Autodesk Fusion 360 part; units mm, degrees
(part 3 of 4)
  point P31 (-40.625, 1.496)
  point P32 (-27.125, 9.2902)
  point P33 (-18.125, 9.2902)
  point P34 (-13.625, 1.496)
  point P35 (-22.625, 1.496)
  point P36 (-9.125, 9.2902)
  point P37 (-0.125, 9.2902)
  point P38 (4.375, 1.496)
  point P39 (-4.625, 1.496)
  point P40 (8.875, 9.2902)
  point P41 (17.875, 9.2902)
  point P42 (22.375, 1.496)
  point P43 (13.375, 1.496)
  point P44 (-153.125, 25.1672)
  point P45 (-144.125, 25.1672)
  point P46 (-139.625, 17.373)
  point P47 (-148.625, 17.373)
  point P48 (-135.125, 25.1672)
  point P49 (-126.125, 25.1672)
  point P50 (-121.625, 17.373)
  point P51 (-130.625, 17.373)
  point P52 (-117.125, 25.1672)
  point P53 (-108.125, 25.1672)
  point P54 (-103.625, 17.373)
  point P55 (-112.625, 17.373)
  point P56 (-99.125, 25.1672)
  point P57 (-90.125, 25.1672)
  point P58 (-85.625, 17.373)
  point P59 (-94.625, 17.373)
  point P60 (-81.125, 25.1672)
  point P61 (-72.125, 25.1672)
  point P62 (-67.625, 17.373)
  point P63 (-76.625, 17.373)
  point P64 (-63.125, 25.1672)
  point P65 (-54.125, 25.1672)
  point P66 (-49.625, 17.373)
  point P67 (-58.625, 17.373)
  point P68 (-45.125, 25.1672)
  point P69 (-36.125, 25.1672)
  point P70 (-31.625, 17.373)
  point P71 (-40.625, 17.373)
  point P72 (-27.125, 25.1672)
  point P73 (-18.125, 25.1672)
  point P74 (-13.625, 17.373)
  point P75 (-22.625, 17.373)
  point P76 (-9.125, 25.1672)
  point P77 (-0.125, 25.1672)
  point P78 (4.375, 17.373)
  point P79 (-4.625, 17.373)
  point P80 (8.875, 25.1672)
  point P81 (17.875, 25.1672)
  point P82 (22.375, 17.373)
  point P83 (13.375, 17.373)
  point P84 (-153.125, 41.0442)
  point P85 (-144.125, 41.0442)
  point P86 (-139.625, 33.25)
  point P87 (-148.625, 33.25)
  point P88 (-135.125, 41.0442)
  point P89 (-126.125, 41.0442)
  point P90 (-121.625, 33.25)
  point P91 (-130.625, 33.25)
  point P92 (-117.125, 41.0442)
  point P93 (-108.125, 41.0442)
  point P94 (-103.625, 33.25)
  point P95 (-112.625, 33.25)
  point P96 (-99.125, 41.0442)
  point P97 (-90.125, 41.0442)
  point P98 (-85.625, 33.25)
  point P99 (-94.625, 33.25)
  point P100 (-63.125, 41.0442)
  point P101 (-54.125, 41.0442)
  point P102 (-49.625, 33.25)
  point P103 (-58.625, 33.25)
  point P104 (-45.125, 41.0442)
  point P105 (-36.125, 41.0442)
  point P106 (-31.625, 33.25)
  point P107 (-40.625, 33.25)
  point P108 (-27.125, 41.0442)
  point P109 (-18.125, 41.0442)
  point P110 (-13.625, 33.25)
  point P111 (-22.625, 33.25)
  point P112 (-9.125, 41.0442)
  point P113 (-0.125, 41.0442)
  point P114 (4.375, 33.25)
  point P115 (-4.625, 33.25)
  point P116 (8.875, 41.0442)
  point P117 (17.875, 41.0442)
  point P118 (22.375, 33.25)
  point P119 (13.375, 33.25)
  point P120 (-153.125, 56.9212)
  point P121 (-144.125, 56.9212)
  point P122 (-139.625, 49.127)
  point P123 (-148.625, 49.127)
  point P124 (-135.125, 56.9212)
  point P125 (-126.125, 56.9212)
  point P126 (-121.625, 49.127)
  point P127 (-130.625, 49.127)
  point P128 (-117.125, 56.9212)
  point P129 (-108.125, 56.9212)
  point P130 (-103.625, 49.127)
  point P131 (-112.625, 49.127)
  point P132 (-99.125, 56.9212)
  point P133 (-90.125, 56.9212)
  point P134 (-85.625, 49.127)
  point P135 (-94.625, 49.127)
  point P136 (-81.125, 56.9212)
  point P137 (-72.125, 56.9212)
  point P138 (-67.625, 49.127)
  point P139 (-76.625, 49.127)
  point P140 (-63.125, 56.9212)
  point P141 (-54.125, 56.9212)
  point P142 (-49.625, 49.127)
  point P143 (-58.625, 49.127)
  point P144 (-45.125, 56.9212)
  point P145 (-36.125, 56.9212)
  point P146 (-31.625, 49.127)
  point P147 (-40.625, 49.127)
  point P148 (-27.125, 56.9212)
  point P149 (-18.125, 56.9212)
  point P150 (-13.625, 49.127)
  point P151 (-22.625, 49.127)
  point P152 (-9.125, 56.9212)
  point P153 (-0.125, 56.9212)
  point P154 (4.375, 49.127)
  point P155 (-4.625, 49.127)
  point P156 (8.875, 56.9212)
  point P157 (17.875, 56.9212)
  point P158 (22.375, 49.127)
  point P159 (13.375, 49.127)
  point P160 (-153.125, 72.7982)
  point P161 (-144.125, 72.7982)
  point P162 (-139.625, 65.004)
  point P163 (-148.625, 65.004)
  point P164 (-135.125, 72.7982)
  point P165 (-126.125, 72.7982)
  point P166 (-121.625, 65.004)
  point P167 (-130.625, 65.004)
  point P168 (-117.125, 72.7982)
  point P169 (-108.125, 72.7982)
  point P170 (-103.625, 65.004)
  point P171 (-112.625, 65.004)
  point P172 (-99.125, 72.7982)
  point P173 (-90.125, 72.7982)
  point P174 (-85.625, 65.004)
  point P175 (-94.625, 65.004)
  point P176 (-81.125, 72.7982)
  point P177 (-72.125, 72.7982)
  point P178 (-67.625, 65.004)
  point P179 (-76.625, 65.004)
  point P180 (-63.125, 72.7982)
  point P181 (-54.125, 72.7982)
  point P182 (-49.625, 65.004)
  point P183 (-58.625, 65.004)
  point P184 (-45.125, 72.7982)
  point P185 (-36.125, 72.7982)
  point P186 (-31.625, 65.004)
  point P187 (-40.625, 65.004)
  point P188 (-27.125, 72.7982)
  point P189 (-18.125, 72.7982)
  point P190 (-13.625, 65.004)
  point P191 (-22.625, 65.004)
  point P192 (-9.125, 72.7982)
  point P193 (-0.125, 72.7982)
  point P194 (4.375, 65.004)
  point P195 (-4.625, 65.004)
  point P196 (8.875, 72.7982)
  point P197 (17.875, 72.7982)
  point P198 (22.375, 65.004)
  point P199 (13.375, 65.004)
  point P200 (-153.125, 88.6752)
  point P201 (-144.125, 88.6752)
  point P202 (-139.625, 80.881)
  point P203 (-148.625, 80.881)
  point P204 (-135.125, 88.6752)
  point P205 (-126.125, 88.6752)
  point P206 (-121.625, 80.881)
  point P207 (-130.625, 80.881)
  point P208 (-117.125, 88.6752)
  point P209 (-108.125, 88.6752)
  point P210 (-103.625, 80.881)
  point P211 (-112.625, 80.881)
  point P212 (-99.125, 88.6752)
  point P213 (-90.125, 88.6752)
  point P214 (-85.625, 80.881)
  point P215 (-94.625, 80.881)
  point P216 (-81.125, 88.6752)
  point P217 (-72.125, 88.6752)
  point P218 (-67.625, 80.881)
  point P219 (-76.625, 80.881)
  point P220 (-63.125, 88.6752)
  point P221 (-54.125, 88.6752)
  point P222 (-49.625, 80.881)
  point P223 (-58.625, 80.881)
  point P224 (-45.125, 88.6752)
  point P225 (-36.125, 88.6752)
  point P226 (-31.625, 80.881)
  point P227 (-40.625, 80.881)
  point P228 (-27.125, 88.6752)
  point P229 (-18.125, 88.6752)
  point P230 (-13.625, 80.881)
  point P231 (-22.625, 80.881)
  point P232 (-9.125, 88.6752)
  point P233 (-0.125, 88.6752)
  point P234 (4.375, 80.881)
  point P235 (-4.625, 80.881)
  point P236 (8.875, 88.6752)
  point P237 (17.875, 88.6752)
  point P238 (22.375, 80.881)
  point P239 (13.375, 80.881)
  dimension "d110" = 2
  dimension "d111" = 150.75
  dimension "d112" = 2
  dimension "d113" = 2
  dimension "d115" = 150.75
  dimension "d116" = 6
  dimension "d118" = 3.5
  dimension "d119" = 3.5
  dimension "d120" = 3.5
  dimension "d121" = 3.5
  dimension "d122" = 2
  dimension "d123" = 2
  dimension "d124" = 2
  dimension "d125" = 2
  dimension "d126" = 2
  dimension "d129" = 18
  dimension "d130" = 15.877
  dimension "d131" = 2
  constraint horizontal L16
  constraint vertical L17
  constraint coincident L11.end L12.start
  constraint horizontal L18
  constraint vertical L19
  constraint horizontal L20
  constraint vertical L21
  constraint horizontal L22
  constraint vertical L23
  constraint horizontal L24
  constraint vertical L25
  constraint horizontal L26
  constraint vertical L27
  constraint vertical L28
  constraint vertical L29
  constraint horizontal L30
  constraint vertical L31
  constraint coincident L19 L29.end
  constraint coincident L14 L29.end
  constraint horizontal L32
  constraint vertical L33
  constraint vertical L34
  constraint horizontal L35
  constraint coincident L12.end L13.start
  constraint horizontal L36
  constraint vertical L37
  constraint horizontal L38
  constraint vertical L39
  constraint coincident L38 L40.end
  constraint perpendicular L38 L40
  constraint horizontal L1481
  constraint vertical L1482
  constraint horizontal L1483
  constraint vertical L1484
  constraint perpendicular L18 L1485
  measures "d110" distance of L17.end L18.end
  measures "d111" distance of L19.end L10.end
  measures "d112" distance of L19.end L24.end
  measures "d113" distance of L23.end L26.end
  measures "d115" distance of L11.end L36.end
  measures "d116" distance of L11.end L38.end
  measures "d118" distance of P0 L46
  measures "d119" distance of P1 L52
  measures "d120" distance of P2 L58
  measures "d121" distance of P3 L64
  measures "d122" distance of L42 L63
  measures "d123" distance of L55 L64
  measures "d124" distance of L41 L56
  measures "d125" distance of L46 L49
  measures "d126" distance of L48 L57
  measures "d131" distance of L29.end L1483.end
extrude "Extrude18" cut sketch "Sketch14" against normal blind 2 contours L38 L263 L264 L267 L268 L269 L272 | L19 L29 L258 L262 L271 L1485 | L38 L233 L234 L235 L238 L247 L249 | L19 L29 L500 L505 L506 L510 L520 | L38 L239 L240 L243 L244 L245 L248 | L19 L29 L498 L502 L511 | L38 L209 L210 L211 L214 L223 L225 | L19 L29 L714 L718 L727 | L19 L29 L716 L721 L722 L726 L736 | L38 L215 L216 L219 L220 L221 L224 | L19 L29 L958 L967 L1483 | L19 L29 L956 L961 L962 L966 L976 | L38 L185 L186 L187 L190 L199 L201 | L960 L964 L965 L968 L1483 | L38 L191 L192 L195 L196 L197 L200 | L931 L934 L943 L945 L1483 | L38 L161 L162 L163 L166 L175 L177 | L936 L940 L941 L944 L1483 | L38 L167 L168 L171 L172 L173 L176 | L907 L910 L919 L921 L1483 | L38 L137 L138 L139 L142 L151 L153 | L912 L916 L917 L920 L1483 | L38 L143 L144 L147 L148 L149 L152 | L883 L886 L895 L897 L1483 | L38 L113 L114 L115 L118 L127 L129 | L27 L31 L40 L72 L75 L77 | L38 L65 L66 L67 L70 L79 L81 | L888 L892 L893 L896 L1483 | L38 L119 L120 L123 L124 L125 L128 | L27 L31 L312 L315 L317 | L27 L31 L309 L313 L314 L318 L328 | L38 L95 L96 L99 L100 L101 L104 | L859 L862 L871 L873 L1483 | L38 L89 L90 L91 L94 L103 L105 | L27 L31 L552 L555 L557 | L27 L31 L549 L553 L554 L558 L568 | L864 L868 L869 L872 L1483 | L27 L31 L768 L773 L1483 | L27 L31 L765 L769 L770 L774 L784 | L835 L838 L847 L849 L1483 | L840 L844 L845 L848 L1483 | L763 L766 L775 L777 L1483 | L811 L814 L823 L825 L1483 | L792 L796 L797 L800 L1483 | L816 L820 L821 L824 L1483 | L787 L790 L799 L801 L1483 | L41 L42 L43 L44 L45 L46 | L47 L48 L49 L50 L51 L52 | L53 L54 L55 L56 L57 L58 | L59 L60 L61 L62 L63 L64 | L305 L306 L307 L310 L319 L321 | L322 L323 L324 L325 L326 L327 | L329 L330 L331 L334 L343 L345 | L332 L333 L337 L338 L342 L352 | L335 L336 L339 L340 L341 L344 | L346 L347 L348 L349 L350 L351 | L353 L354 L355 L358 L367 L369 | L356 L357 L361 L362 L366 L376 | L359 L360 L363 L364 L365 L368 | L370 L371 L372 L373 L374 L375 | L377 L378 L379 L382 L391 L393 | L380 L381 L385 L386 L390 L400 | L383 L384 L387 L388 L389 L392 | L394 L395 L396 L397 L398 L399 | L401 L402 L403 L406 L415 L417 | L404 L405 L409 L410 L414 L424 | L407 L408 L411 L412 L413 L416 | L418 L419 L420 L421 L422 L423 | L425 L426 L427 L430 L439 L441 | L428 L429 L433 L434 L438 L448 | L431 L432 L435 L436 L437 L440 | L442 L443 L444 L445 L446 L447 | L449 L450 L451 L454 L463 L465 | L452 L453 L457 L458 L462 L472 | L455 L456 L459 L460 L461 L464 | L466 L467 L468 L469 L470 L471 | L473 L474 L475 L478 L487 L489 | L476 L477 L481 L482 L486 L496 | L479 L480 L483 L484 L485 L488 | L490 L491 L492 L493 L494 L495 | L503 L504 L507 L508 L509 L512 | L545 L546 L547 L550 L559 L561 | L562 L563 L564 L565 L566 L567 | L569 L570 L571 L574 L583 L585 | L572 L573 L577 L578 L582 L592 | L575 L576 L579 L580 L581 L584 | L586 L587 L588 L589 L590 L591 | L593 L594 L595 L598 L607 L609 | L596 L597 L601 L602 L606 L616 | L599 L600 L603 L604 L605 L608 | L610 L611 L612 L613 L614 L615 | L617 L618 L619 L622 L631 L633 | L620 L621 L625 L626 L630 L640 | L623 L624 L627 L628 L629 L632 | L634 L635 L636 L637 L638 L639 | L641 L642 L643 L646 L655 L657 | L644 L645 L649 L650 L654 L664 | L647 L648 L651 L652 L653 L656 | L658 L659 L660 L661 L662 L663 | L665 L666 L667 L670 L679 L681 | L668 L669 L673 L674 L678 L688 | L671 L672 L675 L676 L677 L680 | L682 L683 L684 L685 L686 L687 | L689 L690 L691 L694 L703 L705 | L692 L693 L697 L698 L702 L712 | L695 L696 L699 L700 L701 L704 | L706 L707 L708 L709 L710 L711 | L719 L720 L723 L724 L725 L728 | L778 L779 L780 L781 L782 L783 | L788 L789 L793 L794 L798 L808 | L802 L803 L804 L805 L806 L807 | L812 L813 L817 L818 L822 L832 | L826 L827 L828 L829 L830 L831 | L836 L837 L841 L842 L846 L856 | L850 L851 L852 L853 L854 L855 | L860 L861 L865 L866 L870 L880 | L874 L875 L876 L877 L878 L879 | L884 L885 L889 L890 L894 L904 | L898 L899 L900 L901 L902 L903 | L908 L909 L913 L914 L918 L928 | L922 L923 L924 L925 L926 L927 | L932 L933 L937 L938 L942 L952 | L946 L947 L948 L949 L950 L951 bodies 2
sketch "Sketch15" plane through (0, 0, 0) normal (1, 0, 0) x (0, 0, -1)
  line L0 (85, 3) -> (85, 3.5)
  arc A0 (86, 4.5) -> (85, 3.5) centre (86, 3.5) ccw
  line L1 (86, 4.5) -> (104, 4.5)
  arc A1 (105, 3.5) -> (104, 4.5) centre (104, 3.5) ccw
  line L2 (105, 3.5) -> (105, 3)
  arc A2 (104, 2) -> (105, 3) centre (104, 3) ccw
  line L3 (104, 2) -> (86, 2)
  arc A3 (85, 3) -> (86, 2) centre (86, 3) ccw
  line L4 (29, 2) -> (11, 2)
  arc A4 (10, 3) -> (11, 2) centre (11, 3) ccw
  line L5 (10, 3) -> (10, 3.5)
  arc A5 (11, 4.5) -> (10, 3.5) centre (11, 3.5) ccw
  line L6 (11, 4.5) -> (29, 4.5)
  arc A6 (30, 3.5) -> (29, 4.5) centre (29, 3.5) ccw
  line L7 (30, 3.5) -> (30, 3)
  arc A7 (29, 2) -> (30, 3) centre (29, 3) ccw
  line L8 (10.25, 71) -> (114.75, 71)
  line L9 (114.75, 71) -> (114.75, 85)
  line L10 (114.75, 85) -> (-2, 85)
  line L11 (-2, 85) -> (-2, 0)
  line L12 (-2, 0) -> (114.75, 0)
  line L13 (114.75, 0) -> (114.75, 60)
  line L14 (114.75, 60) -> (10.25, 60)
  line L15 (10.25, 60) -> (10.25, 71)
  line L16 (114.75, 0) -> (-2, 0)
  line L17 (-2, 0) -> (-2, 6)
  line L18 (-2, 6) -> (114.75, 6)
  line L19 (114.75, 6) -> (114.75, 0)
  line L20 (-2, 6) -> (0, 6)
  line L21 (0, 6) -> (0, 60)
  line L22 (0, 60) -> (-2, 60)
  line L23 (-2, 60) -> (-2, 6)
  line L24 (-2, 60) -> (114.75, 60)
  line L25 (114.75, 60) -> (114.75, 58)
  line L26 (114.75, 58) -> (-2, 58)
  line L27 (-2, 58) -> (-2, 60)
  line L28 (114.75, 58) -> (112.75, 58)
  line L29 (112.75, 58) -> (112.75, 6)
  line L30 (112.75, 6) -> (114.75, 6)
  line L31 (114.75, 6) -> (114.75, 58)
  line L32 (112.75, 32) -> (112.75, 6)
  line L33 (112.75, 6) -> (56.375, 6)
  line L34 (59.875, 34.0207) -> (56.375, 36.0415)
  line L35 (56.375, 36.0415) -> (52.875, 34.0207)
  line L36 (52.875, 34.0207) -> (52.875, 29.9793)
  line L37 (52.875, 29.9793) -> (56.375, 27.9585)
  line L38 (56.375, 27.9585) -> (59.875, 29.9793)
  line L39 (59.875, 29.9793) -> (59.875, 34.0207)
  line L40 (68.875, 34.0207) -> (65.375, 36.0415)
  line L41 (65.375, 36.0415) -> (61.875, 34.0207)
  line L42 (61.875, 34.0207) -> (61.875, 29.9793)
  line L43 (61.875, 29.9793) -> (65.375, 27.9585)
  line L44 (65.375, 27.9585) -> (68.875, 29.9793)
  line L45 (68.875, 29.9793) -> (68.875, 34.0207)
  line L46 (64.375, 41.815) -> (60.875, 43.8357)
  line L47 (60.875, 43.8357) -> (57.375, 41.815)
  line L48 (57.375, 41.815) -> (57.375, 37.7735)
  line L49 (57.375, 37.7735) -> (60.875, 35.7528)
  line L50 (60.875, 35.7528) -> (64.375, 37.7735)
  line L51 (64.375, 37.7735) -> (64.375, 41.815)
  line L52 (55.375, 41.815) -> (51.875, 43.8357)
  line L53 (51.875, 43.8357) -> (48.375, 41.815)
  line L54 (48.375, 41.815) -> (48.375, 37.7735)
  line L55 (48.375, 37.7735) -> (51.875, 35.7528)
  line L56 (51.875, 35.7528) -> (55.375, 37.7735)
  line L57 (55.375, 37.7735) -> (55.375, 41.815)
  line L58 (1.375, 10.061) -> (-2.125, 12.0817)
  line L59 (10.375, 6.0195) -> (10.375, 10.061)
  line L60 (6.875, 12.0817) -> (3.375, 10.061)
  line L61 (3.375, 6.0195) -> (6.875, 3.9988)
  line L62 (5.875, 2.2667) -> (2.375, 4.2875)
  line L63 (1.375, 6.0195) -> (1.375, 10.061)
  line L64 (11.375, -3.7955) -> (14.875, -1.7747)
  line L65 (-5.625, 10.061) -> (-5.625, 6.0195)
  line L66 (6.875, 3.9988) -> (10.375, 6.0195)
  line L67 (2.375, 4.2875) -> (-1.125, 2.2667)
  line L68 (-2.125, 3.9988) -> (1.375, 6.0195)
  line L69 (10.375, 10.061) -> (6.875, 12.0817)
  line L70 (-5.625, 6.0195) -> (-2.125, 3.9988)
  line L71 (2.375, -3.7955) -> (5.875, -1.7747)
  line L72 (11.375, 4.2875) -> (7.875, 2.2667)
  line L73 (3.375, 10.061) -> (3.375, 6.0195)
  line L74 (-1.125, -1.7747) -> (2.375, -3.7955)
  line L75 (7.875, -1.7747) -> (11.375, -3.7955)
  line L76 (7.875, 2.2667) -> (7.875, -1.7747)
  line L77 (5.875, -1.7747) -> (5.875, 2.2667)
  line L78 (-1.125, 2.2667) -> (-1.125, -1.7747)
  line L79 (14.875, -1.7747) -> (14.875, 2.2667)
  line L80 (-2.125, 12.0817) -> (-5.625, 10.061)
  line L81 (14.875, 2.2667) -> (11.375, 4.2875)
  line L82 (19.375, 10.061) -> (15.875, 12.0817)
  line L83 (28.375, 6.0195) -> (28.375, 10.061)
  line L84 (24.875, 12.0817) -> (21.375, 10.061)
  line L85 (21.375, 6.0195) -> (24.875, 3.9988)
  line L86 (23.875, 2.2667) -> (20.375, 4.2875)
  line L87 (19.375, 6.0195) -> (19.375, 10.061)
  line L88 (29.375, -3.7955) -> (32.875, -1.7747)
  line L89 (12.375, 10.061) -> (12.375, 6.0195)
  line L90 (24.875, 3.9988) -> (28.375, 6.0195)
  line L91 (20.375, 4.2875) -> (16.875, 2.2667)
  line L92 (15.875, 3.9988) -> (19.375, 6.0195)
  line L93 (28.375, 10.061) -> (24.875, 12.0817)
  line L94 (12.375, 6.0195) -> (15.875, 3.9988)
  line L95 (20.375, -3.7955) -> (23.875, -1.7747)
  line L96 (29.375, 4.2875) -> (25.875, 2.2667)
  line L97 (21.375, 10.061) -> (21.375, 6.0195)
  line L98 (16.875, -1.7747) -> (20.375, -3.7955)
  line L99 (25.875, -1.7747) -> (29.375, -3.7955)
  line L100 (25.875, 2.2667) -> (25.875, -1.7747)
  line L101 (23.875, -1.7747) -> (23.875, 2.2667)
  line L102 (16.875, 2.2667) -> (16.875, -1.7747)
  line L103 (32.875, -1.7747) -> (32.875, 2.2667)
  line L104 (15.875, 12.0817) -> (12.375, 10.061)
  line L105 (32.875, 2.2667) -> (29.375, 4.2875)
  line L106 (37.375, 10.061) -> (33.875, 12.0817)
  line L107 (46.375, 6.0195) -> (46.375, 10.061)
  line L108 (42.875, 12.0817) -> (39.375, 10.061)
  line L109 (39.375, 6.0195) -> (42.875, 3.9988)
  line L110 (41.875, 2.2667) -> (38.375, 4.2875)
  line L111 (37.375, 6.0195) -> (37.375, 10.061)
  line L112 (47.375, -3.7955) -> (50.875, -1.7747)
  line L113 (30.375, 10.061) -> (30.375, 6.0195)
  line L114 (42.875, 3.9988) -> (46.375, 6.0195)
  line L115 (38.375, 4.2875) -> (34.875, 2.2667)
  line L116 (33.875, 3.9988) -> (37.375, 6.0195)
  line L117 (46.375, 10.061) -> (42.875, 12.0817)
  line L118 (30.375, 6.0195) -> (33.875, 3.9988)
  line L119 (38.375, -3.7955) -> (41.875, -1.7747)
  line L120 (47.375, 4.2875) -> (43.875, 2.2667)
  line L121 (39.375, 10.061) -> (39.375, 6.0195)
  line L122 (34.875, -1.7747) -> (38.375, -3.7955)
  line L123 (43.875, -1.7747) -> (47.375, -3.7955)
  line L124 (43.875, 2.2667) -> (43.875, -1.7747)
  line L125 (41.875, -1.7747) -> (41.875, 2.2667)
  line L126 (34.875, 2.2667) -> (34.875, -1.7747)
  line L127 (50.875, -1.7747) -> (50.875, 2.2667)
  line L128 (33.875, 12.0817) -> (30.375, 10.061)
  line L129 (50.875, 2.2667) -> (47.375, 4.2875)
  line L130 (55.375, 10.061) -> (51.875, 12.0817)
  line L131 (64.375, 6.0195) -> (64.375, 10.061)
  line L132 (60.875, 12.0817) -> (57.375, 10.061)
  line L133 (57.375, 6.0195) -> (60.875, 3.9988)
  line L134 (59.875, 2.2667) -> (56.375, 4.2875)
  line L135 (55.375, 6.0195) -> (55.375, 10.061)
  line L136 (65.375, -3.7955) -> (68.875, -1.7747)
  line L137 (48.375, 10.061) -> (48.375, 6.0195)
  line L138 (60.875, 3.9988) -> (64.375, 6.0195)
  line L139 (56.375, 4.2875) -> (52.875, 2.2667)
  line L140 (51.875, 3.9988) -> (55.375, 6.0195)
  line L141 (64.375, 10.061) -> (60.875, 12.0817)
  line L142 (48.375, 6.0195) -> (51.875, 3.9988)
  line L143 (56.375, -3.7955) -> (59.875, -1.7747)
  line L144 (65.375, 4.2875) -> (61.875, 2.2667)
  line L145 (57.375, 10.061) -> (57.375, 6.0195)
  line L146 (52.875, -1.7747) -> (56.375, -3.7955)
  line L147 (61.875, -1.7747) -> (65.375, -3.7955)
  line L148 (61.875, 2.2667) -> (61.875, -1.7747)
  line L149 (59.875, -1.7747) -> (59.875, 2.2667)
  line L150 (52.875, 2.2667) -> (52.875, -1.7747)
  line L151 (68.875, -1.7747) -> (68.875, 2.2667)
  line L152 (51.875, 12.0817) -> (48.375, 10.061)
  line L153 (68.875, 2.2667) -> (65.375, 4.2875)
  line L154 (73.375, 10.061) -> (69.875, 12.0817)
  line L155 (82.375, 6.0195) -> (82.375, 10.061)
  line L156 (78.875, 12.0817) -> (75.375, 10.061)
  line L157 (75.375, 6.0195) -> (78.875, 3.9988)
  line L158 (77.875, 2.2667) -> (74.375, 4.2875)
  line L159 (73.375, 6.0195) -> (73.375, 10.061)
  line L160 (83.375, -3.7955) -> (86.875, -1.7747)
  line L161 (66.375, 10.061) -> (66.375, 6.0195)
  line L162 (78.875, 3.9988) -> (82.375, 6.0195)
  line L163 (74.375, 4.2875) -> (70.875, 2.2667)
  line L164 (69.875, 3.9988) -> (73.375, 6.0195)
  line L165 (82.375, 10.061) -> (78.875, 12.0817)
  line L166 (66.375, 6.0195) -> (69.875, 3.9988)
  line L167 (74.375, -3.7955) -> (77.875, -1.7747)
  line L168 (83.375, 4.2875) -> (79.875, 2.2667)
  line L169 (75.375, 10.061) -> (75.375, 6.0195)
  line L170 (70.875, -1.7747) -> (74.375, -3.7955)
  line L171 (79.875, -1.7747) -> (83.375, -3.7955)
  line L172 (79.875, 2.2667) -> (79.875, -1.7747)
  line L173 (77.875, -1.7747) -> (77.875, 2.2667)
  line L174 (70.875, 2.2667) -> (70.875, -1.7747)
  line L175 (86.875, -1.7747) -> (86.875, 2.2667)
  line L176 (69.875, 12.0817) -> (66.375, 10.061)
  line L177 (86.875, 2.2667) -> (83.375, 4.2875)
  line L178 (91.375, 10.061) -> (87.875, 12.0817)
  line L179 (100.375, 6.0195) -> (100.375, 10.061)
  line L180 (96.875, 12.0817) -> (93.375, 10.061)
  line L181 (93.375, 6.0195) -> (96.875, 3.9988)
  line L182 (95.875, 2.2667) -> (92.375, 4.2875)
  line L183 (91.375, 6.0195) -> (91.375, 10.061)
  line L184 (101.375, -3.7955) -> (104.875, -1.7747)
  line L185 (84.375, 10.061) -> (84.375, 6.0195)
  line L186 (96.875, 3.9988) -> (100.375, 6.0195)
  line L187 (92.375, 4.2875) -> (88.875, 2.2667)
  line L188 (87.875, 3.9988) -> (91.375, 6.0195)
  line L189 (100.375, 10.061) -> (96.875, 12.0817)
  line L190 (84.375, 6.0195) -> (87.875, 3.9988)
  line L191 (92.375, -3.7955) -> (95.875, -1.7747)
  line L192 (101.375, 4.2875) -> (97.875, 2.2667)
  line L193 (93.375, 10.061) -> (93.375, 6.0195)
  line L194 (88.875, -1.7747) -> (92.375, -3.7955)
  line L195 (97.875, -1.7747) -> (101.375, -3.7955)
  line L196 (97.875, 2.2667) -> (97.875, -1.7747)
  line L197 (95.875, -1.7747) -> (95.875, 2.2667)
  line L198 (88.875, 2.2667) -> (88.875, -1.7747)
  line L199 (104.875, -1.7747) -> (104.875, 2.2667)
  line L200 (87.875, 12.0817) -> (84.375, 10.061)
  line L201 (104.875, 2.2667) -> (101.375, 4.2875)
  line L202 (109.375, 10.061) -> (105.875, 12.0817)
  line L203 (118.375, 6.0195) -> (118.375, 10.061)
  line L204 (114.875, 12.0817) -> (111.375, 10.061)
  line L205 (111.375, 6.0195) -> (114.875, 3.9988)
  line L206 (113.875, 2.2667) -> (110.375, 4.2875)
  line L207 (109.375, 6.0195) -> (109.375, 10.061)
  line L208 (119.375, -3.7955) -> (122.875, -1.7747)
  line L209 (102.375, 10.061) -> (102.375, 6.0195)
  line L210 (114.875, 3.9988) -> (118.375, 6.0195)
  line L211 (110.375, 4.2875) -> (106.875, 2.2667)
  line L212 (105.875, 3.9988) -> (109.375, 6.0195)
  line L213 (118.375, 10.061) -> (114.875, 12.0817)
  line L214 (102.375, 6.0195) -> (105.875, 3.9988)
  line L215 (110.375, -3.7955) -> (113.875, -1.7747)
  line L216 (119.375, 4.2875) -> (115.875, 2.2667)
  line L217 (111.375, 10.061) -> (111.375, 6.0195)
  line L218 (106.875, -1.7747) -> (110.375, -3.7955)
  line L219 (115.875, -1.7747) -> (119.375, -3.7955)
  line L220 (115.875, 2.2667) -> (115.875, -1.7747)
  line L221 (113.875, -1.7747) -> (113.875, 2.2667)
  line L222 (106.875, 2.2667) -> (106.875, -1.7747)
  line L223 (122.875, -1.7747) -> (122.875, 2.2667)
  line L224 (105.875, 12.0817) -> (102.375, 10.061)
  line L225 (122.875, 2.2667) -> (119.375, 4.2875)
  line L226 (1.375, 25.938) -> (-2.125, 27.9587)
  line L227 (10.375, 21.8965) -> (10.375, 25.938)
  line L228 (6.875, 27.9587) -> (3.375, 25.938)
  line L229 (3.375, 21.8965) -> (6.875, 19.8758)
  line L230 (5.875, 18.1437) -> (2.375, 20.1645)
  line L231 (1.375, 21.8965) -> (1.375, 25.938)
  line L232 (11.375, 12.0815) -> (14.875, 14.1023)
  line L233 (-5.625, 25.938) -> (-5.625, 21.8965)
  line L234 (6.875, 19.8758) -> (10.375, 21.8965)
  line L235 (2.375, 20.1645) -> (-1.125, 18.1437)
  line L236 (-2.125, 19.8758) -> (1.375, 21.8965)
  line L237 (10.375, 25.938) -> (6.875, 27.9587)
  line L238 (-5.625, 21.8965) -> (-2.125, 19.8758)
  line L239 (2.375, 12.0815) -> (5.875, 14.1023)
  line L240 (11.375, 20.1645) -> (7.875, 18.1437)
  line L241 (3.375, 25.938) -> (3.375, 21.8965)
  line L242 (-1.125, 14.1023) -> (2.375, 12.0815)
  line L243 (7.875, 14.1023) -> (11.375, 12.0815)
  line L244 (7.875, 18.1437) -> (7.875, 14.1023)
  line L245 (5.875, 14.1023) -> (5.875, 18.1437)
  line L246 (-1.125, 18.1437) -> (-1.125, 14.1023)
  line L247 (14.875, 14.1023) -> (14.875, 18.1437)
  line L248 (-2.125, 27.9587) -> (-5.625, 25.938)
  line L249 (14.875, 18.1437) -> (11.375, 20.1645)
  line L250 (19.375, 25.938) -> (15.875, 27.9587)
  line L251 (28.375, 21.8965) -> (28.375, 25.938)
  line L252 (24.875, 27.9587) -> (21.375, 25.938)
  line L253 (21.375, 21.8965) -> (24.875, 19.8758)
  line L254 (23.875, 18.1437) -> (20.375, 20.1645)
  line L255 (19.375, 21.8965) -> (19.375, 25.938)
  line L256 (29.375, 12.0815) -> (32.875, 14.1023)
  line L257 (12.375, 25.938) -> (12.375, 21.8965)
  line L258 (24.875, 19.8758) -> (28.375, 21.8965)
  line L259 (20.375, 20.1645) -> (16.875, 18.1437)
  line L260 (15.875, 19.8758) -> (19.375, 21.8965)
  line L261 (28.375, 25.938) -> (24.875, 27.9587)
  line L262 (12.375, 21.8965) -> (15.875, 19.8758)
  line L263 (20.375, 12.0815) -> (23.875, 14.1023)
  line L264 (29.375, 20.1645) -> (25.875, 18.1437)
  line L265 (21.375, 25.938) -> (21.375, 21.8965)
  line L266 (16.875, 14.1023) -> (20.375, 12.0815)
  line L267 (25.875, 14.1023) -> (29.375, 12.0815)
  line L268 (25.875, 18.1437) -> (25.875, 14.1023)
  line L269 (23.875, 14.1023) -> (23.875, 18.1437)
  line L270 (16.875, 18.1437) -> (16.875, 14.1023)
  line L271 (32.875, 14.1023) -> (32.875, 18.1437)
  line L272 (15.875, 27.9587) -> (12.375, 25.938)
  line L273 (32.875, 18.1437) -> (29.375, 20.1645)
  line L274 (37.375, 25.938) -> (33.875, 27.9587)
  line L275 (46.375, 21.8965) -> (46.375, 25.938)
  line L276 (42.875, 27.9587) -> (39.375, 25.938)
  line L277 (39.375, 21.8965) -> (42.875, 19.8758)
  line L278 (41.875, 18.1437) -> (38.375, 20.1645)
  line L279 (37.375, 21.8965) -> (37.375, 25.938)
  line L280 (47.375, 12.0815) -> (50.875, 14.1023)
  line L281 (30.375, 25.938) -> (30.375, 21.8965)
  line L282 (42.875, 19.8758) -> (46.375, 21.8965)
  line L283 (38.375, 20.1645) -> (34.875, 18.1437)
  line L284 (33.875, 19.8758) -> (37.375, 21.8965)
  line L285 (46.375, 25.938) -> (42.875, 27.9587)
  line L286 (30.375, 21.8965) -> (33.875, 19.8758)
  line L287 (38.375, 12.0815) -> (41.875, 14.1023)
  line L288 (47.375, 20.1645) -> (43.875, 18.1437)
  line L289 (39.375, 25.938) -> (39.375, 21.8965)
  line L290 (34.875, 14.1023) -> (38.375, 12.0815)
  line L291 (43.875, 14.1023) -> (47.375, 12.0815)
  line L292 (43.875, 18.1437) -> (43.875, 14.1023)
  line L293 (41.875, 14.1023) -> (41.875, 18.1437)
  line L294 (34.875, 18.1437) -> (34.875, 14.1023)
  line L295 (50.875, 14.1023) -> (50.875, 18.1437)
  line L296 (33.875, 27.9587) -> (30.375, 25.938)
  line L297 (50.875, 18.1437) -> (47.375, 20.1645)
  line L298 (55.375, 25.938) -> (51.875, 27.9587)
  line L299 (64.375, 21.8965) -> (64.375, 25.938)
  line L300 (60.875, 27.9587) -> (57.375, 25.938)
  line L301 (57.375, 21.8965) -> (60.875, 19.8758)
  line L302 (59.875, 18.1437) -> (56.375, 20.1645)
  line L303 (55.375, 21.8965) -> (55.375, 25.938)
  line L304 (65.375, 12.0815) -> (68.875, 14.1023)
  line L305 (48.375, 25.938) -> (48.375, 21.8965)
  line L306 (60.875, 19.8758) -> (64.375, 21.8965)
  line L307 (56.375, 20.1645) -> (52.875, 18.1437)
  line L308 (51.875, 19.8758) -> (55.375, 21.8965)
  line L309 (64.375, 25.938) -> (60.875, 27.9587)
  line L310 (48.375, 21.8965) -> (51.875, 19.8758)
  line L311 (56.375, 12.0815) -> (59.875, 14.1023)
  line L312 (65.375, 20.1645) -> (61.875, 18.1437)
  line L313 (57.375, 25.938) -> (57.375, 21.8965)
  line L314 (52.875, 14.1023) -> (56.375, 12.0815)
  line L315 (61.875, 14.1023) -> (65.375, 12.0815)
  line L316 (61.875, 18.1437) -> (61.875, 14.1023)
  line L317 (59.875, 14.1023) -> (59.875, 18.1437)
  line L318 (52.875, 18.1437) -> (52.875, 14.1023)
  line L319 (68.875, 14.1023) -> (68.875, 18.1437)
  line L320 (51.875, 27.9587) -> (48.375, 25.938)
  line L321 (68.875, 18.1437) -> (65.375, 20.1645)
  line L322 (73.375, 25.938) -> (69.875, 27.9587)
  line L323 (82.375, 21.8965) -> (82.375, 25.938)
  line L324 (78.875, 27.9587) -> (75.375, 25.938)
  line L325 (75.375, 21.8965) -> (78.875, 19.8758)
  line L326 (77.875, 18.1437) -> (74.375, 20.1645)
  line L327 (73.375, 21.8965) -> (73.375, 25.938)
  line L328 (83.375, 12.0815) -> (86.875, 14.1023)
  line L329 (66.375, 25.938) -> (66.375, 21.8965)
  line L330 (78.875, 19.8758) -> (82.375, 21.8965)
  line L331 (74.375, 20.1645) -> (70.875, 18.1437)
  line L332 (69.875, 19.8758) -> (73.375, 21.8965)
  line L333 (82.375, 25.938) -> (78.875, 27.9587)
  line L334 (66.375, 21.8965) -> (69.875, 19.8758)
  line L335 (74.375, 12.0815) -> (77.875, 14.1023)
  line L336 (83.375, 20.1645) -> (79.875, 18.1437)
  line L337 (75.375, 25.938) -> (75.375, 21.8965)
  line L338 (70.875, 14.1023) -> (74.375, 12.0815)
  line L339 (79.875, 14.1023) -> (83.375, 12.0815)
  line L340 (79.875, 18.1437) -> (79.875, 14.1023)
  line L341 (77.875, 14.1023) -> (77.875, 18.1437)
  line L342 (70.875, 18.1437) -> (70.875, 14.1023)
  line L343 (86.875, 14.1023) -> (86.875, 18.1437)
  line L344 (69.875, 27.9587) -> (66.375, 25.938)
  line L345 (86.875, 18.1437) -> (83.375, 20.1645)
  line L346 (91.375, 25.938) -> (87.875, 27.9587)
  line L347 (100.375, 21.8965) -> (100.375, 25.938)
  line L348 (96.875, 27.9587) -> (93.375, 25.938)
  line L349 (93.375, 21.8965) -> (96.875, 19.8758)
  line L350 (95.875, 18.1437) -> (92.375, 20.1645)
  line L351 (91.375, 21.8965) -> (91.375, 25.938)
  line L352 (101.375, 12.0815) -> (104.875, 14.1023)
  line L353 (84.375, 25.938) -> (84.375, 21.8965)
  line L354 (96.875, 19.8758) -> (100.375, 21.8965)
  line L355 (92.375, 20.1645) -> (88.875, 18.1437)
  line L356 (87.875, 19.8758) -> (91.375, 21.8965)
  line L357 (100.375, 25.938) -> (96.875, 27.9587)
  line L358 (84.375, 21.8965) -> (87.875, 19.8758)
  line L359 (92.375, 12.0815) -> (95.875, 14.1023)
  line L360 (101.375, 20.1645) -> (97.875, 18.1437)
  line L361 (93.375, 25.938) -> (93.375, 21.8965)
  line L362 (88.875, 14.1023) -> (92.375, 12.0815)
  line L363 (97.875, 14.1023) -> (101.375, 12.0815)
  line L364 (97.875, 18.1437) -> (97.875, 14.1023)
  line L365 (95.875, 14.1023) -> (95.875, 18.1437)
  line L366 (88.875, 18.1437) -> (88.875, 14.1023)
  line L367 (104.875, 14.1023) -> (104.875, 18.1437)
  line L368 (87.875, 27.9587) -> (84.375, 25.938)
  line L369 (104.875, 18.1437) -> (101.375, 20.1645)
  line L370 (109.375, 25.938) -> (105.875, 27.9587)
  line L371 (118.375, 21.8965) -> (118.375, 25.938)
  line L372 (114.875, 27.9587) -> (111.375, 25.938)
  line L373 (111.375, 21.8965) -> (114.875, 19.8758)
  line L374 (113.875, 18.1437) -> (110.375, 20.1645)
  line L375 (109.375, 21.8965) -> (109.375, 25.938)
  line L376 (119.375, 12.0815) -> (122.875, 14.1023)
  line L377 (102.375, 25.938) -> (102.375, 21.8965)
  line L378 (114.875, 19.8758) -> (118.375, 21.8965)
  line L379 (110.375, 20.1645) -> (106.875, 18.1437)
  line L380 (105.875, 19.8758) -> (109.375, 21.8965)
  line L381 (118.375, 25.938) -> (114.875, 27.9587)
  line L382 (102.375, 21.8965) -> (105.875, 19.8758)
  line L383 (110.375, 12.0815) -> (113.875, 14.1023)
  line L384 (119.375, 20.1645) -> (115.875, 18.1437)
  line L385 (111.375, 25.938) -> (111.375, 21.8965)
  line L386 (106.875, 14.1023) -> (110.375, 12.0815)
  line L387 (115.875, 14.1023) -> (119.375, 12.0815)
  line L388 (115.875, 18.1437) -> (115.875, 14.1023)
  line L389 (113.875, 14.1023) -> (113.875, 18.1437)
  line L390 (106.875, 18.1437) -> (106.875, 14.1023)
  line L391 (122.875, 14.1023) -> (122.875, 18.1437)
  line L392 (105.875, 27.9587) -> (102.375, 25.938)
  line L393 (122.875, 18.1437) -> (119.375, 20.1645)
  line L394 (1.375, 41.815) -> (-2.125, 43.8357)
  line L395 (10.375, 37.7735) -> (10.375, 41.815)
  line L396 (6.875, 43.8357) -> (3.375, 41.815)
  line L397 (3.375, 37.7735) -> (6.875, 35.7528)
  line L398 (5.875, 34.0207) -> (2.375, 36.0415)
  line L399 (1.375, 37.7735) -> (1.375, 41.815)
  line L400 (11.375, 27.9585) -> (14.875, 29.9793)
  line L401 (-5.625, 41.815) -> (-5.625, 37.7735)
  line L402 (6.875, 35.7528) -> (10.375, 37.7735)
  line L403 (2.375, 36.0415) -> (-1.125, 34.0207)
  line L404 (-2.125, 35.7528) -> (1.375, 37.7735)
  line L405 (10.375, 41.815) -> (6.875, 43.8357)
  line L406 (-5.625, 37.7735) -> (-2.125, 35.7528)
  line L407 (2.375, 27.9585) -> (5.875, 29.9793)
  line L408 (11.375, 36.0415) -> (7.875, 34.0207)
  line L409 (3.375, 41.815) -> (3.375, 37.7735)
  line L410 (-1.125, 29.9793) -> (2.375, 27.9585)
  line L411 (7.875, 29.9793) -> (11.375, 27.9585)
  line L412 (7.875, 34.0207) -> (7.875, 29.9793)
  line L413 (5.875, 29.9793) -> (5.875, 34.0207)
  line L414 (-1.125, 34.0207) -> (-1.125, 29.9793)
  line L415 (14.875, 29.9793) -> (14.875, 34.0207)
  line L416 (-2.125, 43.8357) -> (-5.625, 41.815)
  line L417 (14.875, 34.0207) -> (11.375, 36.0415)
  line L418 (19.375, 41.815) -> (15.875, 43.8357)
  line L419 (28.375, 37.7735) -> (28.375, 41.815)
  line L420 (24.875, 43.8357) -> (21.375, 41.815)
  line L421 (21.375, 37.7735) -> (24.875, 35.7528)
  line L422 (23.875, 34.0207) -> (20.375, 36.0415)
  line L423 (19.375, 37.7735) -> (19.375, 41.815)
  line L424 (29.375, 27.9585) -> (32.875, 29.9793)
  line L425 (12.375, 41.815) -> (12.375, 37.7735)
  line L426 (24.875, 35.7528) -> (28.375, 37.7735)
  line L427 (20.375, 36.0415) -> (16.875, 34.0207)
  line L428 (15.875, 35.7528) -> (19.375, 37.7735)
  line L429 (28.375, 41.815) -> (24.875, 43.8357)
  line L430 (12.375, 37.7735) -> (15.875, 35.7528)
  line L431 (20.375, 27.9585) -> (23.875, 29.9793)
  line L432 (29.375, 36.0415) -> (25.875, 34.0207)
  line L433 (21.375, 41.815) -> (21.375, 37.7735)
  line L434 (16.875, 29.9793) -> (20.375, 27.9585)
  line L435 (25.875, 29.9793) -> (29.375, 27.9585)
  line L436 (25.875, 34.0207) -> (25.875, 29.9793)
  line L437 (23.875, 29.9793) -> (23.875, 34.0207)
  line L438 (16.875, 34.0207) -> (16.875, 29.9793)
  line L439 (32.875, 29.9793) -> (32.875, 34.0207)
  line L440 (15.875, 43.8357) -> (12.375, 41.815)
  line L441 (32.875, 34.0207) -> (29.375, 36.0415)
  line L442 (37.375, 41.815) -> (33.875, 43.8357)
  line L443 (46.375, 37.7735) -> (46.375, 41.815)
  line L444 (42.875, 43.8357) -> (39.375, 41.815)
  line L445 (39.375, 37.7735) -> (42.875, 35.7528)
  line L446 (41.875, 34.0207) -> (38.375, 36.0415)
  line L447 (37.375, 37.7735) -> (37.375, 41.815)
  line L448 (47.375, 27.9585) -> (50.875, 29.9793)
  line L449 (30.375, 41.815) -> (30.375, 37.7735)
  line L450 (42.875, 35.7528) -> (46.375, 37.7735)
  line L451 (38.375, 36.0415) -> (34.875, 34.0207)
  line L452 (33.875, 35.7528) -> (37.375, 37.7735)
  line L453 (46.375, 41.815) -> (42.875, 43.8357)
  line L454 (30.375, 37.7735) -> (33.875, 35.7528)
  line L455 (38.375, 27.9585) -> (41.875, 29.9793)
  line L456 (47.375, 36.0415) -> (43.875, 34.0207)
  line L457 (39.375, 41.815) -> (39.375, 37.7735)
  line L458 (34.875, 29.9793) -> (38.375, 27.9585)
  line L459 (43.875, 29.9793) -> (47.375, 27.9585)
  line L460 (43.875, 34.0207) -> (43.875, 29.9793)
  line L461 (41.875, 29.9793) -> (41.875, 34.0207)
  line L462 (34.875, 34.0207) -> (34.875, 29.9793)
  line L463 (50.875, 29.9793) -> (50.875, 34.0207)
  line L464 (33.875, 43.8357) -> (30.375, 41.815)
  line L465 (50.875, 34.0207) -> (47.375, 36.0415)
  line L466 (73.375, 41.815) -> (69.875, 43.8357)
  line L467 (82.375, 37.7735) -> (82.375, 41.815)
  line L468 (78.875, 43.8357) -> (75.375, 41.815)
  line L469 (75.375, 37.7735) -> (78.875, 35.7528)
  line L470 (77.875, 34.0207) -> (74.375, 36.0415)
  line L471 (73.375, 37.7735) -> (73.375, 41.815)
  line L472 (83.375, 27.9585) -> (86.875, 29.9793)
  line L473 (66.375, 41.815) -> (66.375, 37.7735)
  line L474 (78.875, 35.7528) -> (82.375, 37.7735)
  line L475 (74.375, 36.0415) -> (70.875, 34.0207)
  line L476 (69.875, 35.7528) -> (73.375, 37.7735)
  line L477 (82.375, 41.815) -> (78.875, 43.8357)
  line L478 (66.375, 37.7735) -> (69.875, 35.7528)
  line L479 (74.375, 27.9585) -> (77.875, 29.9793)
  line L480 (83.375, 36.0415) -> (79.875, 34.0207)
  line L481 (75.375, 41.815) -> (75.375, 37.7735)
  line L482 (70.875, 29.9793) -> (74.375, 27.9585)
  line L483 (79.875, 29.9793) -> (83.375, 27.9585)
  line L484 (79.875, 34.0207) -> (79.875, 29.9793)
  line L485 (77.875, 29.9793) -> (77.875, 34.0207)
  line L486 (70.875, 34.0207) -> (70.875, 29.9793)
  line L487 (86.875, 29.9793) -> (86.875, 34.0207)
  line L488 (69.875, 43.8357) -> (66.375, 41.815)
  line L489 (86.875, 34.0207) -> (83.375, 36.0415)
  line L490 (91.375, 41.815) -> (87.875, 43.8357)
  line L491 (100.375, 37.7735) -> (100.375, 41.815)
  line L492 (96.875, 43.8357) -> (93.375, 41.815)
  line L493 (93.375, 37.7735) -> (96.875, 35.7528)
  line L494 (95.875, 34.0207) -> (92.375, 36.0415)
  line L495 (91.375, 37.7735) -> (91.375, 41.815)
  line L496 (101.375, 27.9585) -> (104.875, 29.9793)
  line L497 (84.375, 41.815) -> (84.375, 37.7735)
  line L498 (96.875, 35.7528) -> (100.375, 37.7735)
  line L499 (92.375, 36.0415) -> (88.875, 34.0207)
  line L500 (87.875, 35.7528) -> (91.375, 37.7735)
  line L501 (100.375, 41.815) -> (96.875, 43.8357)
  line L502 (84.375, 37.7735) -> (87.875, 35.7528)
  line L503 (92.375, 27.9585) -> (95.875, 29.9793)
  line L504 (101.375, 36.0415) -> (97.875, 34.0207)
  line L505 (93.375, 41.815) -> (93.375, 37.7735)
  line L506 (88.875, 29.9793) -> (92.375, 27.9585)
  line L507 (97.875, 29.9793) -> (101.375, 27.9585)
  line L508 (97.875, 34.0207) -> (97.875, 29.9793)
  line L509 (95.875, 29.9793) -> (95.875, 34.0207)
  line L510 (88.875, 34.0207) -> (88.875, 29.9793)
  line L511 (104.875, 29.9793) -> (104.875, 34.0207)
  line L512 (87.875, 43.8357) -> (84.375, 41.815)
  line L513 (104.875, 34.0207) -> (101.375, 36.0415)
  line L514 (109.375, 41.815) -> (105.875, 43.8357)
  line L515 (118.375, 37.7735) -> (118.375, 41.815)
  line L516 (114.875, 43.8357) -> (111.375, 41.815)
  line L517 (111.375, 37.7735) -> (114.875, 35.7528)
  line L518 (113.875, 34.0207) -> (110.375, 36.0415)
  line L519 (109.375, 37.7735) -> (109.375, 41.815)
  line L520 (119.375, 27.9585) -> (122.875, 29.9793)
  line L521 (102.375, 41.815) -> (102.375, 37.7735)
  line L522 (114.875, 35.7528) -> (118.375, 37.7735)
  line L523 (110.375, 36.0415) -> (106.875, 34.0207)
  line L524 (105.875, 35.7528) -> (109.375, 37.7735)
  line L525 (118.375, 41.815) -> (114.875, 43.8357)
  line L526 (102.375, 37.7735) -> (105.875, 35.7528)
  line L527 (110.375, 27.9585) -> (113.875, 29.9793)
  line L528 (119.375, 36.0415) -> (115.875, 34.0207)
  line L529 (111.375, 41.815) -> (111.375, 37.7735)
  line L530 (106.875, 29.9793) -> (110.375, 27.9585)
  line L531 (115.875, 29.9793) -> (119.375, 27.9585)
  line L532 (115.875, 34.0207) -> (115.875, 29.9793)
  line L533 (113.875, 29.9793) -> (113.875, 34.0207)
  line L534 (106.875, 34.0207) -> (106.875, 29.9793)
  line L535 (122.875, 29.9793) -> (122.875, 34.0207)
  line L536 (105.875, 43.8357) -> (102.375, 41.815)
  line L537 (122.875, 34.0207) -> (119.375, 36.0415)
  line L538 (1.375, 57.692) -> (-2.125, 59.7127)
  line L539 (10.375, 53.6505) -> (10.375, 57.692)
  line L540 (6.875, 59.7127) -> (3.375, 57.692)
  line L541 (3.375, 53.6505) -> (6.875, 51.6298)
  line L542 (5.875, 49.8977) -> (2.375, 51.9185)
  line L543 (1.375, 53.6505) -> (1.375, 57.692)
  line L544 (11.375, 43.8355) -> (14.875, 45.8563)
  line L545 (-5.625, 57.692) -> (-5.625, 53.6505)
  line L546 (6.875, 51.6298) -> (10.375, 53.6505)
  line L547 (2.375, 51.9185) -> (-1.125, 49.8977)
  line L548 (-2.125, 51.6298) -> (1.375, 53.6505)
  line L549 (10.375, 57.692) -> (6.875, 59.7127)
  line L550 (-5.625, 53.6505) -> (-2.125, 51.6298)
  line L551 (2.375, 43.8355) -> (5.875, 45.8563)
  line L552 (11.375, 51.9185) -> (7.875, 49.8977)
  line L553 (3.375, 57.692) -> (3.375, 53.6505)
  line L554 (-1.125, 45.8563) -> (2.375, 43.8355)
  line L555 (7.875, 45.8563) -> (11.375, 43.8355)
  line L556 (7.875, 49.8977) -> (7.875, 45.8563)
  line L557 (5.875, 45.8563) -> (5.875, 49.8977)
  line L558 (-1.125, 49.8977) -> (-1.125, 45.8563)
  line L559 (14.875, 45.8563) -> (14.875, 49.8977)
  line L560 (-2.125, 59.7127) -> (-5.625, 57.692)
  line L561 (14.875, 49.8977) -> (11.375, 51.9185)
  line L562 (19.375, 57.692) -> (15.875, 59.7127)
  line L563 (28.375, 53.6505) -> (28.375, 57.692)
  line L564 (24.875, 59.7127) -> (21.375, 57.692)
  line L565 (21.375, 53.6505) -> (24.875, 51.6298)
  line L566 (23.875, 49.8977) -> (20.375, 51.9185)
  line L567 (19.375, 53.6505) -> (19.375, 57.692)
  line L568 (29.375, 43.8355) -> (32.875, 45.8563)
  line L569 (12.375, 57.692) -> (12.375, 53.6505)
  line L570 (24.875, 51.6298) -> (28.375, 53.6505)
  line L571 (20.375, 51.9185) -> (16.875, 49.8977)
  line L572 (15.875, 51.6298) -> (19.375, 53.6505)
  line L573 (28.375, 57.692) -> (24.875, 59.7127)
  line L574 (12.375, 53.6505) -> (15.875, 51.6298)
  line L575 (20.375, 43.8355) -> (23.875, 45.8563)
  line L576 (29.375, 51.9185) -> (25.875, 49.8977)
  line L577 (21.375, 57.692) -> (21.375, 53.6505)
  line L578 (16.875, 45.8563) -> (20.375, 43.8355)
  line L579 (25.875, 45.8563) -> (29.375, 43.8355)
  line L580 (25.875, 49.8977) -> (25.875, 45.8563)
  line L581 (23.875, 45.8563) -> (23.875, 49.8977)
  line L582 (16.875, 49.8977) -> (16.875, 45.8563)
  line L583 (32.875, 45.8563) -> (32.875, 49.8977)
  line L584 (15.875, 59.7127) -> (12.375, 57.692)
  line L585 (32.875, 49.8977) -> (29.375, 51.9185)
  line L586 (37.375, 57.692) -> (33.875, 59.7127)
  line L587 (46.375, 53.6505) -> (46.375, 57.692)
  line L588 (42.875, 59.7127) -> (39.375, 57.692)
  line L589 (39.375, 53.6505) -> (42.875, 51.6298)
  line L590 (41.875, 49.8977) -> (38.375, 51.9185)
  line L591 (37.375, 53.6505) -> (37.375, 57.692)
  line L592 (47.375, 43.8355) -> (50.875, 45.8563)
  line L593 (30.375, 57.692) -> (30.375, 53.6505)
  line L594 (42.875, 51.6298) -> (46.375, 53.6505)
  line L595 (38.375, 51.9185) -> (34.875, 49.8977)
  line L596 (33.875, 51.6298) -> (37.375, 53.6505)
  line L597 (46.375, 57.692) -> (42.875, 59.7127)
  line L598 (30.375, 53.6505) -> (33.875, 51.6298)
  line L599 (38.375, 43.8355) -> (41.875, 45.8563)
  line L600 (47.375, 51.9185) -> (43.875, 49.8977)
  line L601 (39.375, 57.692) -> (39.375, 53.6505)
  line L602 (34.875, 45.8563) -> (38.375, 43.8355)
  line L603 (43.875, 45.8563) -> (47.375, 43.8355)
  line L604 (43.875, 49.8977) -> (43.875, 45.8563)
  line L605 (41.875, 45.8563) -> (41.875, 49.8977)
  line L606 (34.875, 49.8977) -> (34.875, 45.8563)
  line L607 (50.875, 45.8563) -> (50.875, 49.8977)
  line L608 (33.875, 59.7127) -> (30.375, 57.692)
  line L609 (50.875, 49.8977) -> (47.375, 51.9185)
  line L610 (55.375, 57.692) -> (51.875, 59.7127)
  line L611 (64.375, 53.6505) -> (64.375, 57.692)
  line L612 (60.875, 59.7127) -> (57.375, 57.692)
  line L613 (57.375, 53.6505) -> (60.875, 51.6298)
  line L614 (59.875, 49.8977) -> (56.375, 51.9185)
  line L615 (55.375, 53.6505) -> (55.375, 57.692)
  line L616 (65.375, 43.8355) -> (68.875, 45.8563)
  line L617 (48.375, 57.692) -> (48.375, 53.6505)
  line L618 (60.875, 51.6298) -> (64.375, 53.6505)
  line L619 (56.375, 51.9185) -> (52.875, 49.8977)
  line L620 (51.875, 51.6298) -> (55.375, 53.6505)
  line L621 (64.375, 57.692) -> (60.875, 59.7127)
  line L622 (48.375, 53.6505) -> (51.875, 51.6298)
  line L623 (56.375, 43.8355) -> (59.875, 45.8563)
  line L624 (65.375, 51.9185) -> (61.875, 49.8977)
  line L625 (57.375, 57.692) -> (57.375, 53.6505)
  line L626 (52.875, 45.8563) -> (56.375, 43.8355)
  line L627 (61.875, 45.8563) -> (65.375, 43.8355)
  line L628 (61.875, 49.8977) -> (61.875, 45.8563)
  line L629 (59.875, 45.8563) -> (59.875, 49.8977)
  line L630 (52.875, 49.8977) -> (52.875, 45.8563)
  line L631 (68.875, 45.8563) -> (68.875, 49.8977)
  line L632 (51.875, 59.7127) -> (48.375, 57.692)
  line L633 (68.875, 49.8977) -> (65.375, 51.9185)
  line L634 (73.375, 57.692) -> (69.875, 59.7127)
  line L635 (82.375, 53.6505) -> (82.375, 57.692)
  line L636 (78.875, 59.7127) -> (75.375, 57.692)
  line L637 (75.375, 53.6505) -> (78.875, 51.6298)
  line L638 (77.875, 49.8977) -> (74.375, 51.9185)
  line L639 (73.375, 53.6505) -> (73.375, 57.692)
  line L640 (83.375, 43.8355) -> (86.875, 45.8563)
  line L641 (66.375, 57.692) -> (66.375, 53.6505)
  line L642 (78.875, 51.6298) -> (82.375, 53.6505)
  line L643 (74.375, 51.9185) -> (70.875, 49.8977)
  line L644 (69.875, 51.6298) -> (73.375, 53.6505)
  line L645 (82.375, 57.692) -> (78.875, 59.7127)
  line L646 (66.375, 53.6505) -> (69.875, 51.6298)
  line L647 (74.375, 43.8355) -> (77.875, 45.8563)
  line L648 (83.375, 51.9185) -> (79.875, 49.8977)
  line L649 (75.375, 57.692) -> (75.375, 53.6505)
  line L650 (70.875, 45.8563) -> (74.375, 43.8355)
  line L651 (79.875, 45.8563) -> (83.375, 43.8355)
  line L652 (79.875, 49.8977) -> (79.875, 45.8563)
  line L653 (77.875, 45.8563) -> (77.875, 49.8977)
  line L654 (70.875, 49.8977) -> (70.875, 45.8563)
  line L655 (86.875, 45.8563) -> (86.875, 49.8977)
  line L656 (69.875, 59.7127) -> (66.375, 57.692)
  line L657 (86.875, 49.8977) -> (83.375, 51.9185)
  line L658 (91.375, 57.692) -> (87.875, 59.7127)
  line L659 (100.375, 53.6505) -> (100.375, 57.692)
  line L660 (96.875, 59.7127) -> (93.375, 57.692)
  line L661 (93.375, 53.6505) -> (96.875, 51.6298)
  line L662 (95.875, 49.8977) -> (92.375, 51.9185)
  line L663 (91.375, 53.6505) -> (91.375, 57.692)
  line L664 (101.375, 43.8355) -> (104.875, 45.8563)
  line L665 (84.375, 57.692) -> (84.375, 53.6505)
  line L666 (96.875, 51.6298) -> (100.375, 53.6505)
  line L667 (92.375, 51.9185) -> (88.875, 49.8977)
  line L668 (87.875, 51.6298) -> (91.375, 53.6505)
  line L669 (100.375, 57.692) -> (96.875, 59.7127)
  line L670 (84.375, 53.6505) -> (87.875, 51.6298)
  line L671 (92.375, 43.8355) -> (95.875, 45.8563)
  line L672 (101.375, 51.9185) -> (97.875, 49.8977)
  line L673 (93.375, 57.692) -> (93.375, 53.6505)
  line L674 (88.875, 45.8563) -> (92.375, 43.8355)
  line L675 (97.875, 45.8563) -> (101.375, 43.8355)
  line L676 (97.875, 49.8977) -> (97.875, 45.8563)
  line L677 (95.875, 45.8563) -> (95.875, 49.8977)
  line L678 (88.875, 49.8977) -> (88.875, 45.8563)
  line L679 (104.875, 45.8563) -> (104.875, 49.8977)
  line L680 (87.875, 59.7127) -> (84.375, 57.692)
  line L681 (104.875, 49.8977) -> (101.375, 51.9185)
  line L682 (109.375, 57.692) -> (105.875, 59.7127)
  line L683 (118.375, 53.6505) -> (118.375, 57.692)
  line L684 (114.875, 59.7127) -> (111.375, 57.692)
  line L685 (111.375, 53.6505) -> (114.875, 51.6298)
  line L686 (113.875, 49.8977) -> (110.375, 51.9185)
  line L687 (109.375, 53.6505) -> (109.375, 57.692)
  line L688 (119.375, 43.8355) -> (122.875, 45.8563)
  line L689 (102.375, 57.692) -> (102.375, 53.6505)
  line L690 (114.875, 51.6298) -> (118.375, 53.6505)
  line L691 (110.375, 51.9185) -> (106.875, 49.8977)
  line L692 (105.875, 51.6298) -> (109.375, 53.6505)
  line L693 (118.375, 57.692) -> (114.875, 59.7127)
  line L694 (102.375, 53.6505) -> (105.875, 51.6298)
  line L695 (110.375, 43.8355) -> (113.875, 45.8563)
  line L696 (119.375, 51.9185) -> (115.875, 49.8977)
  line L697 (111.375, 57.692) -> (111.375, 53.6505)
  line L698 (106.875, 45.8563) -> (110.375, 43.8355)
  line L699 (115.875, 45.8563) -> (119.375, 43.8355)
  line L700 (115.875, 49.8977) -> (115.875, 45.8563)
  line L701 (113.875, 45.8563) -> (113.875, 49.8977)
  line L702 (106.875, 49.8977) -> (106.875, 45.8563)
  line L703 (122.875, 45.8563) -> (122.875, 49.8977)
  line L704 (105.875, 59.7127) -> (102.375, 57.692)
  line L705 (122.875, 49.8977) -> (119.375, 51.9185)
  line L706 (1.375, 73.569) -> (-2.125, 75.5897)
  line L707 (10.375, 69.5275) -> (10.375, 73.569)
  line L708 (6.875, 75.5897) -> (3.375, 73.569)
  line L709 (3.375, 69.5275) -> (6.875, 67.5068)
  line L710 (5.875, 65.7747) -> (2.375, 67.7955)
  line L711 (1.375, 69.5275) -> (1.375, 73.569)
  line L712 (11.375, 59.7125) -> (14.875, 61.7333)
  line L713 (-5.625, 73.569) -> (-5.625, 69.5275)
  line L714 (6.875, 67.5068) -> (10.375, 69.5275)
  line L715 (2.375, 67.7955) -> (-1.125, 65.7747)
  line L716 (-2.125, 67.5068) -> (1.375, 69.5275)
  line L717 (10.375, 73.569) -> (6.875, 75.5897)
  line L718 (-5.625, 69.5275) -> (-2.125, 67.5068)
  line L719 (2.375, 59.7125) -> (5.875, 61.7333)
  line L720 (11.375, 67.7955) -> (7.875, 65.7747)
  line L721 (3.375, 73.569) -> (3.375, 69.5275)
  line L722 (-1.125, 61.7333) -> (2.375, 59.7125)
  line L723 (7.875, 61.7333) -> (11.375, 59.7125)
  line L724 (7.875, 65.7747) -> (7.875, 61.7333)
  line L725 (5.875, 61.7333) -> (5.875, 65.7747)
  line L726 (-1.125, 65.7747) -> (-1.125, 61.7333)
  line L727 (14.875, 61.7333) -> (14.875, 65.7747)
  line L728 (-2.125, 75.5897) -> (-5.625, 73.569)
  line L729 (14.875, 65.7747) -> (11.375, 67.7955)
  line L730 (19.375, 73.569) -> (15.875, 75.5897)
  line L731 (28.375, 69.5275) -> (28.375, 73.569)
  line L732 (24.875, 75.5897) -> (21.375, 73.569)
  line L733 (21.375, 69.5275) -> (24.875, 67.5068)
  line L734 (23.875, 65.7747) -> (20.375, 67.7955)
  line L735 (19.375, 69.5275) -> (19.375, 73.569)
  line L736 (29.375, 59.7125) -> (32.875, 61.7333)
  line L737 (12.375, 73.569) -> (12.375, 69.5275)
  line L738 (24.875, 67.5068) -> (28.375, 69.5275)
  line L739 (20.375, 67.7955) -> (16.875, 65.7747)